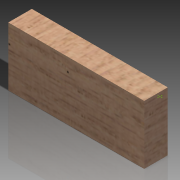
# Autodesk Inventor part: Seitenteil_links_rechts
Saved by Autodesk Inventor 2014 SP1 (Build 180222100, 222)
## iProperties
Created: 2017-12-30
Part Number: Seitenteil_links_rechts
Material: Eiche, weiß
Document SubType Name: Modeling
Designer: Flo
Density: 0.721 g/cm^3
Appearance: Weißeiche - massiv - natur - mittlerer Glanz
Mass: 60.737 g
Surface Area: 147.24 cm^2
Volume: 84.24 cm^3
Author: Flo
Autodesk Inventor part; units mm, degrees
ref_plane "YZ Plane" through (0, 0, 0) normal (1, 0, 0) x (0, 1, 0)
ref_plane "XZ Plane" through (0, 0, 0) normal (0, 1, 0) x (-1, 0, 0)
ref_plane "XY Plane" through (0, 0, 0) normal (0, 0, 1) x (1, 0, 0)
sketch "Skizze1" plane through (0, 0, 0) normal (0, 1, 0) x (-1, 0, 0)
  line L0 (0, 0) -> (104, 0)
  line L1 (104, 0) -> (104, 45)
  line L2 (104, 45) -> (0, 45)
  line L3 (0, 45) -> (0, 0)
  dimension "d0" = 104
  dimension "d1" = 45
  constraints: 8 end point, 2 parallel, 1 horizontal, 1 perpendicular
  measures "d0" distance of L1.end L2.end
  measures "d1" distance of L0.end L1.end
extrude "Extrusion1" add sketch "Skizze1" along normal blind 18
sketch "Skizze2" plane through (-104, 0, 45) normal (0, 0, 1) x (1, 0, 0)
  point P0 (107, 9)
sketch "Skizze3" plane through (-104, 0, 45) normal (0, 0, 1) x (1, 0, 0)
  point P0 (107, 9)
